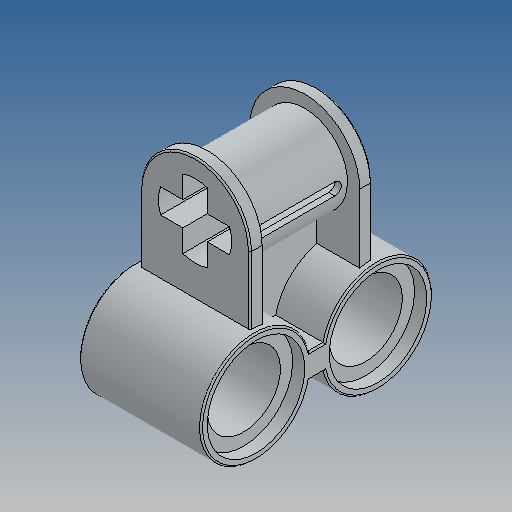
# Autodesk Inventor part: 32291-LtBluishGray
Saved by Autodesk Inventor 2025 (Build 290162010, 162A)
## iProperties
Created: 2014-07-08
Part Number: 32291-LtBluishGray
Material: ABS Plastic
Document SubType Name: Modeling
Designer: D. Kohfeld
Mass: 0.524051 g
Surface Area: 11.1044 cm^2
Volume: 0.494387 cm^3
Density: 1.06 g/cm^3
Appearance: LtBluishGray
Author: D. Kohfeld
Autodesk Inventor part; units mm, degrees
ref_plane "YZ Plane" through (0, 0, 0) normal (1, 0, 0) x (0, 1, 0)
ref_plane "XZ Plane" through (0, 0, 0) normal (0, 1, 0) x (-1, 0, 0)
sketch "Sketch2" plane through (0, 0, 0) normal (1, 0, 0) x (0, 1, 0)
  circle A0 centre (0, 4) radius 3.6
  circle A1 centre (0, -4) radius 3.6
  line L0 (0, 4) -> (0, -4) construction
  line L1 (0.8, 0.49) -> (0.8, -0.49)
  line L2 (-0.8, 0.49) -> (-0.8, -0.49)
  point P0 (0, 0)
  point P1 (0, 0)
  dimension "d0" = 7.2
  dimension "d1" = 1.6
  dimension "d2" = 8
  constraints: 6 end point, 4 point on circle, 3 parallel, 2 centre point, 1 coincident, 1 equal radius, 1 midpoint, 1 vertical
  measures "d0" diameter of A0
  measures "d1" distance between parallel lines of L1 L2
  measures "d2" distance of L0.end L0.start
extrude "Extrusion1" add sketch "Sketch2" along normal mid plane 8
ref_plane "Work Plane2" through (0, 0, 4) normal (0, 0, 1) x (1, 0, 0)
sketch "Sketch4" plane through (0, 0, 0) normal (0, 0, 1) x (1, 0, 0)
  line L0 (-4, 0.8) -> (4, 0.8) projected
  line L1 (-0.8, 0.8) -> (-0.8, 5.3167)
  line L2 (0.8, 0.8) -> (0.8, 5.3167)
  arc A0 (0.8, 5.3167) -> (-0.8, 5.3167) centre (0, 8) ccw
  circle A1 centre (0, 8) radius 2.4 construction
  line L3 (-0.8, 10.2627) -> (-0.8, 8.8)
  line L4 (-0.8, 8.8) -> (-2.2627, 8.8)
  line L5 (-2.2627, 7.2) -> (-0.8, 7.2)
  line L6 (-0.8, 7.2) -> (-0.8, 5.7373)
  line L7 (0.8, 5.7373) -> (0.8, 7.2)
  line L8 (0.8, 7.2) -> (2.2627, 7.2)
  line L9 (2.2627, 8.8) -> (0.8, 8.8)
  line L10 (0.8, 8.8) -> (0.8, 10.2627)
  arc A2 (0.8, 10.2627) -> (-0.8, 10.2627) centre (0, 8) ccw
  arc A3 (-2.2627, 8.8) -> (-2.2627, 7.2) centre (0, 8) ccw
  arc A4 (-0.8, 5.7373) -> (0.8, 5.7373) centre (0, 8) ccw
  arc A5 (2.2627, 7.2) -> (2.2627, 8.8) centre (0, 8) ccw
  point P0 (0, 0)
  dimension "d18" = 4.8
  dimension "d12" = 5.6
  dimension "d14" = 1.6
  dimension "d20" = 1.6
  dimension "d40" = 8
  constraints: 20 end point, 10 point on circle, 8 equal length, 5 centre point, 5 perpendicular, 4 parallel, 2 point on line, 1 coincident, 1 vertical alignment, 14 other
  measures "d12" diameter of A0
  measures "d14" distance between parallel lines of L1 L2
  measures "d20" distance between parallel lines of L10 L3
  measures "d40" distance of A0.centre point (0, 0)
extrude "Extrusion2" add sketch "Sketch4" along normal mid plane 8
sketch "Sketch5" plane through (0, 0, 0) normal (1, 0, 0) x (0, 1, 0)
  line L0 (7.2, 4) -> (8.8, 4) projected
  line L1 (8.8, -4) -> (8.8, 4) projected
  line L2 (7.6, 2.4) -> (7.6, -2.4)
  arc A0 (7.6, -2.4) -> (8.4, -2.4) centre (8, -2.4) ccw
  line L3 (8.4, -2.4) -> (8.4, 2.4)
  arc A1 (8.4, 2.4) -> (7.6, 2.4) centre (8, 2.4) ccw
  point P0 (0, 0)
  point P1 (8, 4)
  point P2 (8.4, 0)
  point P3 (8.8, 0)
  dimension "d23" = 0.8
  dimension "d24" = 5.6
  constraints: 4 end point, 4 point on circle, 4 tangent, 3 midpoint, 2 centre point, 2 parallel, 1 horizontal alignment, 1 vertical alignment
  measures "d23" distance between parallel lines of L2 L3
extrude "Extrusion3" cut sketch "Sketch5" along normal through all both and the other way through all
sketch "Sketch6" plane through (0, 0, 4) normal (0, 0, 1) x (1, 0, 0)
  arc A0 (0.8, 5.3167) -> (-0.8, 5.3167) centre (0, 8) ccw projected
  arc A1 (-2.2627, 8.8) -> (-2.2627, 7.2) centre (0, 8) ccw projected
  line L0 (-0.8, 3.6) -> (0.8, 3.6) projected
  line L1 (3.6, 3.2) -> (3.6, 8)
  arc A2 (3.6, 8) -> (-3.6, 8) centre (0, 8) ccw
  line L2 (-3.6, 8) -> (-3.6, 3.2)
  line L3 (-3.6, 3.2) -> (3.6, 3.2)
  arc A3 (-2.2627, 8.8) -> (-2.2627, 7.2) centre (0, 8) ccw projected
  line L4 (-0.8, 8.8) -> (-2.2627, 8.8) projected
  line L5 (-0.8, 10.2627) -> (-0.8, 8.8) projected
  arc A4 (0.8, 10.2627) -> (-0.8, 10.2627) centre (0, 8) ccw projected
  line L6 (0.8, 8.8) -> (0.8, 10.2627) projected
  line L7 (2.2627, 8.8) -> (0.8, 8.8) projected
  arc A5 (2.2627, 7.2) -> (2.2627, 8.8) centre (0, 8) ccw projected
  line L8 (0.8, 7.2) -> (2.2627, 7.2) projected
  line L9 (0.8, 5.7373) -> (0.8, 7.2) projected
  arc A6 (-0.8, 5.7373) -> (0.8, 5.7373) centre (0, 8) ccw projected
  line L10 (-0.8, 7.2) -> (-0.8, 5.7373) projected
  line L11 (-2.2627, 7.2) -> (-0.8, 7.2) projected
  point P0 (0, 0)
  dimension "d41" = 7.2
  dimension "d42" = 6.4
  constraints: 6 end point, 2 perpendicular, 2 point on circle, 2 tangent, 1 centre point, 1 concentric, 1 parallel
  measures "d41" diameter of A2
  measures "d42" diameter of point (0, 0) L3
extrude "Extrusion4" add sketch "Sketch6" against normal blind 0.8
sketch "Sketch3" plane through (0, 0, 4) normal (0, 0, 1) x (1, 0, 0)
  line L0 (-5.6, 0) -> (5.6, 0) projected
  line L1 (-4, 3.2) -> (-3.2, 3.2)
  line L2 (-3.2, 3.2) -> (-3.2, 2.4)
  line L3 (-3.2, 2.4) -> (3.2, 2.4)
  line L4 (3.2, 2.4) -> (3.2, 3.2)
  line L5 (3.2, 3.2) -> (4, 3.2)
  line L6 (4, 3.2) -> (4, 0)
  line L7 (-4, 0) -> (-4, 3.2)
  line L8 (-4, 0) -> (4, 0)
  line L9 (-4, 3.6) -> (-4, -3.6) projected
  line L10 (4, -3.6) -> (4, 3.6) projected
  point P0 (0, 0)
  point P1 (-4, -0.8)
  point P2 (-4, 0.8)
  point P3 (4, 0.8)
  point P4 (4, -0.8)
  dimension "d7" = 4.8
  dimension "d8" = 6.4
  dimension "d9" = 0.8
  constraints: 16 end point, 4 parallel, 4 point on line, 2 collinear, 2 equal length, 2 perpendicular
  measures "d7" diameter of L3 L0
  measures "d8" diameter of L5 L0
  measures "d9" distance between parallel lines of L10 L4
revolve "Revolution1" cut sketch "Sketch3" angle 360 about axis through (-4, 0, 4) along (1, 0, 0)
mirror "Mirror1" about plane through (0, 0, 0) normal (0, 0, 1) of "Revolution1", "Extrusion4"
fillet "Fillet1" radius 0.1 14 edges at (4, 0, -7.6) (4, 0, 7.6) (-4, 0, 7.6) (4, 0.8, 0) (4, -0.8, 0) (-4, 0, -7.6) (-4, 0.8, 0) (-4, -0.8, 0) (-3.6, 5.8, 4) (3.6, 5.8, 4) (0, 11.6, 4) (-3.6, 5.8, -4) (3.6, 5.8, -4) (0, 11.6, -4)
equation "\"d0\" = tlad"
equation "\"d2\" = lu"
equation "\"d3\" = lu"
equation "\"d18\" = kd"
equation "\"d14\" = wall"
equation "\"d20\" = axlet"
equation "\"d40\" = lu"
equation "\"d21\" = lu"
equation "\"d23\" = tpnw"
equation "\"d41\" = tlad"
equation "\"d42\" = tsd"
equation "\"d29\" = tsl"
equation "\"d7\" = kd"
equation "\"d8\" = tsd"
equation "\"d9\" = tsl"
equation "\"d39\" = lf"
equation "\"tlad\" = 7.2"
equation "\"lu\" = 8"
equation "\"kd\" = 4.8"
equation "\"wall\" = 1.6"
equation "\"axlet\" = 1.6"
equation "\"tpnw\" = 0.8"
equation "\"tsl\" = 0.8"
equation "\"tsd\" = 6.4"
equation "\"lf\" = 0.1"
body "Solid1"
